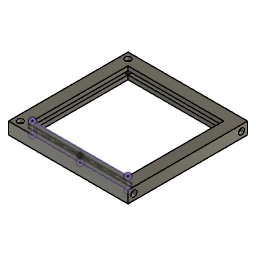
Panel (Autodesk Fusion 360 design; units mm, degrees)
Autodesk Fusion 360 part; units mm, degrees
sketch "Sketch1" plane through (0, 0, 0) normal (0, 0, 1) x (1, 0, 0)
  line L0 (50, 50) -> (-50, 50)
  line L1 (-50, 50) -> (-50, -50)
  line L2 (-50, -50) -> (50, -50)
  line L3 (50, -50) -> (50, 50)
  line L4 (50, 50) -> (-50, -50) construction
  line L5 (-50, 50) -> (50, -50) construction
  line L6 (40, -40) -> (-40, -40)
  line L7 (-40, -40) -> (-40, 40)
  line L8 (-40, 40) -> (40, 40)
  line L9 (40, 40) -> (40, -40)
  line L10 (40, -40) -> (-40, 40) construction
  line L11 (-40, -40) -> (40, 40) construction
  dimension "d1" = 100
  dimension "d2" = 100
  dimension "d3" = 80
  dimension "d4" = 80
  constraint horizontal L0
  constraint perpendicular L0 L1
  constraint parallel L0 L2
  constraint parallel L1 L3
  constraint coincident L4 origin
  constraint coincident L5 origin
  constraint horizontal L6
  constraint perpendicular L6 L7
  constraint parallel L6 L8
  constraint parallel L7 L9
  constraint coincident L10 origin
  constraint coincident L11 origin
  measures "d1" distance of L1.end L2.end
  measures "d2" distance of L0.end L1.end
  measures "d3" distance of L7.end L8.end
  measures "d4" distance of L6.end L7.end
extrude "Extrude1" add sketch "Sketch1" along normal blind 10
sketch "Sketch2" plane through (0, -40, 0) normal (0, 1, 0) x (-1, 0, 0)
  line L0 (-40, 0) -> (40, 0)
  line L1 (40, 0) -> (40, 10)
  line L2 (40, 10) -> (-40, 10)
  line L3 (-40, 10) -> (-40, 0)
  line L4 (0, 10) -> (0, 0) construction
  line L5 (-40, 5) -> (40, 5) construction
  line L6 (43, 3.5) -> (-43, 3.5)
  line L7 (-43, 3.5) -> (-43, 6.5)
  line L8 (-43, 6.5) -> (43, 6.5)
  line L9 (43, 6.5) -> (43, 3.5)
  line L10 (43, 3.5) -> (-43, 6.5) construction
  line L11 (-43, 3.5) -> (43, 6.5) construction
  point P0 (0, 5)
  dimension "d9" = 86
  dimension "d10" = 3
  constraint midpoint L2 L4.start
  constraint coincident L4.end origin
  constraint midpoint L3 L5.start
  constraint midpoint L1 L5.end
  constraint horizontal L6
  constraint perpendicular L6 L7
  constraint parallel L6 L8
  constraint parallel L7 L9
  constraint coincident L10 P0
  constraint coincident L11 P0
  constraint midpoint L4 P0
  measures "d9" distance of L7.end L8.end
  measures "d10" distance of L6.end L7.end
extrude "Extrude2" cut sketch "Sketch2" along normal blind 85 and the other way blind 5 contours L1 L3 L6 L8
extrude "Extrude3" cut sketch "Sketch2" along normal blind 80 contours L3 L6 L7 L8 | L1 L6 L8 L9
sketch "Sketch3" plane through (0, 0, 10) normal (0, 0, 1) x (-1, 0, 0)
  line L0 (40, -40) -> (-40, -40)
  line L1 (-40, -40) -> (-40, 40)
  line L2 (-40, 40) -> (40, 40)
  line L3 (40, 40) -> (40, -40)
  line L4 (-50, 50) -> (-50, -50)
  line L5 (-50, -50) -> (50, -50)
  line L6 (50, -50) -> (50, 50)
  line L7 (50, 50) -> (-50, 50)
  line L8 (40, -40) -> (40, -50) construction
  line L9 (40, -40) -> (50, -40) construction
  line L10 (45, -40) -> (45, -50) construction
  line L11 (40, -45) -> (50, -45) construction
  circle A0 centre (45, -45) radius 2.5
  circle A1 centre (45, 45) radius 2.5
  dimension "d17" = 5
  dimension "d20" = -90
  dimension "d21" = 90
  constraint coincident L0.start L3.end
  constraint coincident L5 L8.end
  constraint perpendicular L5 L8
  constraint coincident L6 L9.end
  constraint perpendicular L6 L9
  constraint midpoint L9 L10.start
  constraint coincident L5 L10.end
  constraint perpendicular L5 L10
  constraint midpoint L8 L11.start
  constraint coincident L6 L11.end
  constraint perpendicular L6 L11
  constraint midpoint L11 A0.centre
  measures "d17" diameter of A0
extrude "Extrude4" cut sketch "Sketch3" against normal blind 3 contours A0 | A1
sketch "Sketch4" plane through (50, 0, 0) normal (1, 0, 0) x (0, 1, 0)
  line L0 (-50, 0) -> (50, 0)
  line L1 (50, 0) -> (50, 10)
  line L2 (50, 10) -> (-50, 10)
  line L3 (-50, 10) -> (-50, 0)
  line L4 (-40, 3.5) -> (-40, 6.5)
  line L5 (-40, 5) -> (-50, 5) construction
  circle A0 centre (-45, 5) radius 2.5
  circle A1 centre (0, 5) radius 2.5
  circle A2 centre (45, 5) radius 2.5
  dimension "d24" = 5
  dimension "d27" = 90
  dimension "d28" = 0
  constraint midpoint L4 L5.start
  constraint midpoint L3 L5.end
  constraint midpoint L5 A0.centre
  measures "d24" diameter of A0
extrude "Extrude5" cut sketch "Sketch4" against normal blind 3 contours A0 | A2
equation "d9 = 80 mm + 6 mm"
equation "d30 = f8e7f7a2-a6e5-415b-bf69-f4a3084041c5"
